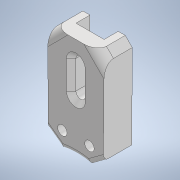
# Autodesk Inventor part: arm_linkage_3
Saved by Autodesk Inventor 2020 (Build 240168000, 168)
## iProperties
Created: 2019-10-19
Part Number: arm_linkage_3
Material: Generic
Document SubType Name: Modeling
Designer: psrob
Density: 1 g/cm^3
Appearance: Default
Author: psrob
Autodesk Inventor part; units mm, degrees
ref_plane "YZ Plane" through (0, 0, 0) normal (1, 0, 0) x (0, 1, 0)
ref_plane "XZ Plane" through (0, 0, 0) normal (0, 1, 0) x (-1, 0, 0)
ref_plane "XY Plane" through (0, 0, 0) normal (0, 0, 1) x (1, 0, 0)
sketch "Sketch1" plane through (0, 0, 0) normal (0, 0, 1) x (1, 0, 0)
  circle A0 centre (2.8817, -5.5305) radius 1 projected
  circle A1 centre (-2.8817, -5.5305) radius 1 projected
  line L0 (4.5, 12.6443) -> (5.9902, 11.1443) projected
  line L1 (3, 12.6443) -> (4.5, 12.6443) projected
  line L2 (3, -2.3557) -> (3, 12.6443) projected
  line L3 (-3, -2.3557) -> (3, -2.3557) projected
  line L4 (-3, 12.6443) -> (-3, -2.3557) projected
  line L5 (-4.5, 12.6443) -> (-3, 12.6443) projected
  line L6 (-5.9902, 11.1443) -> (-4.5, 12.6443) projected
  line L7 (-5.8406, -11.8556) -> (-5.9902, 11.1443) projected
  line L8 (-3.8536, -9.8557) -> (-5.8406, -11.8556) projected
  line L9 (-3.8536, -9.8557) -> (3.8536, -9.8557) projected
  line L10 (5.8406, -11.8556) -> (3.8536, -9.8557) projected
  line L11 (5.9902, 11.1443) -> (5.8406, -11.8556) projected
  line L12 (3.8536, -9.8557) -> (5.8536, -9.8557)
  line L13 (-3.8536, -9.8557) -> (-5.8535, -9.8687)
  point P0 (0, 0)
  constraints: 4 end point, 2 point on line, 1 horizontal, 1 perpendicular
extrude "Extrusion1" add sketch "Sketch1" along normal blind 3 contours L0 L11 L12 L9 L13 L7 L6 L5 L4 L3 L2 L1
sketch "Sketch2" plane through (0, 0, 3) normal (0, 0, 1) x (1, 0, 0)
  line L0 (-3, -2.3557) -> (-3, 12.6443) projected
  line L1 (-3, 12.6443) -> (-4.5, 12.6443) projected
  line L2 (-4.5, 12.6443) -> (-5.9902, 11.1443) projected
  line L3 (-5.9902, 11.1443) -> (-5.8535, -9.8687) projected
  line L4 (-5.8535, -9.8687) -> (-3.8536, -9.8557) projected
  line L5 (-3.8536, -9.8557) -> (5.8536, -9.8557) projected
  line L6 (5.8536, -9.8557) -> (5.9902, 11.1443) projected
  line L7 (5.9902, 11.1443) -> (4.5, 12.6443) projected
  line L8 (4.5, 12.6443) -> (3, 12.6443) projected
  line L9 (3, 12.6443) -> (3, -2.3557) projected
  line L10 (3, -2.3557) -> (-3, -2.3557) projected
  circle A0 centre (-2.8817, -5.5305) radius 1 projected
  circle A1 centre (2.8817, -5.5305) radius 1 projected
  line L11 (3, 12.6443) -> (3, -2.3557) projected
  line L12 (-3, 12.6443) -> (3, 12.6443)
  point P0 (0, 0)
  constraints: 2 end point, 1 horizontal
extrude "Extrusion2" add sketch "Sketch2" along normal blind 3
sketch "Sketch3" plane through (0, 0, 6) normal (0, 0, 1) x (1, 0, 0)
  line L0 (-5.8535, -9.8687) -> (-3.8536, -9.8557) projected
  line L1 (-3.8536, -9.8557) -> (5.8536, -9.8557) projected
  line L2 (5.8536, -9.8557) -> (5.9902, 11.1443) projected
  line L3 (5.9902, 11.1443) -> (4.5, 12.6443) projected
  line L4 (4.5, 12.6443) -> (-4.5, 12.6443) projected
  line L5 (-4.5, 12.6443) -> (-5.9902, 11.1443) projected
  line L6 (-5.9902, 11.1443) -> (-5.8535, -9.8687) projected
  circle A0 centre (2.8817, -5.5305) radius 1 projected
  circle A1 centre (-2.8817, -5.5305) radius 1 projected
  line L7 (-5.8535, -9.8687) -> (-3.8536, -9.8557) projected
  arc A2 (5.8536, -9.8557) -> (-5.8535, -9.8687) centre (0.0154, -23.6729) ccw
  point P0 (0, 0)
  dimension "d4" = 15
  constraints: 2 point on circle, 1 centre point
  measures "d4" radius of A2
extrude "Extrusion3" cut sketch "Sketch3" against normal blind 8 contours A2 L1 L0
chamfer "Chamfer1" distance 3 angle 45 2 edges at (5.8536, -9.8557, 3) (-5.8535, -9.8687, 3)
fillet "Fillet1" radius 2 2 edges at (5.2451, 11.8943, 6) (-5.2451, 11.8943, 6)
fillet "Fillet2" radius 1 3 edges at (-4.4311, -7.9228, 6) (-0.0013, -8.6729, 6) (4.4302, -7.913, 6)
sketch "Sketch4" plane through (0, 0, 6) normal (0, 0, 1) x (1, 0, 0)
  line L0 (-1, 8.1443) -> (-1, 2.1443) projected
  arc A0 (-1, 2.1443) -> (1, 2.1443) centre (0, 2.1443) ccw projected
  line L1 (1, 2.1443) -> (1, 8.1443) projected
  arc A1 (1, 8.1443) -> (-1, 8.1443) centre (0, 8.1443) ccw projected
  line L2 (5.9719, 8.3251) -> (1.6807, 12.6443) projected
  line L3 (5.9719, 8.3251) -> (5.8537, -9.8477) projected
  line L4 (3.4979, -11.4182) -> (5.8537, -9.8477) projected
  spline S0 degree 3 poles (3.7471, -14.0453) (3.5143, -13.7817) (3.313, -13.4738) (3.0785, -12.9028) (3.0205, -12.6553) (3.011, -12.2509) (3.0346, -12.0815) (3.1344, -11.8203) (3.188, -11.725) (3.325, -11.5531) (3.4063, -11.4793) (3.4979, -11.4182) knots 0 0 0 0 0.105501 0.105501 0.185956 0.185956 0.244407 0.244407 0.282215 0.282215 0.320119 0.320119 0.320119 0.320119 projected
  arc A2 (-3.7471, -14.0453) -> (3.7471, -14.0453) centre (0, -17.3557) ccw projected
  spline S1 degree 3 poles (-3.4979, -11.4182) (-3.3811, -11.4961) (-3.2816, -11.5944) (-3.1273, -11.8263) (-3.0754, -11.9539) (-3.0096, -12.2519) (-3.0068, -12.4209) (-3.0565, -12.825) (-3.1338, -13.0604) (-3.3668, -13.5541) (-3.5446, -13.816) (-3.7471, -14.0453) knots 0 0 0 0 0.042129 0.042129 0.083567 0.083567 0.133564 0.133564 0.205298 0.205298 0.296261 0.296261 0.296261 0.296261 projected
  line L5 (-5.8537, -9.8477) -> (-3.4979, -11.4182) projected
  line L6 (-5.8537, -9.8477) -> (-5.9719, 8.3251) projected
  line L7 (-1.6807, 12.6443) -> (-5.9719, 8.3251) projected
  line L8 (-1.6807, 12.6443) -> (1.6807, 12.6443) projected
  circle A3 centre (0, -17.3557) radius 1.5 projected
  circle A4 centre (-2.8817, -5.5305) radius 1 projected
  circle A5 centre (2.8817, -5.5305) radius 1 projected
  point P0 (0, 0)
extrude "Extrusion4" cut sketch "Sketch4" against normal blind 8 contours A1 L1 A0 L0
chamfer "Chamfer2" distance 1 angle 45 4 edges at (-1, 5.1443, 6) (0, 9.1443, 6) (1, 5.1443, 6) (0, 1.1443, 6)
body "Solid1"
